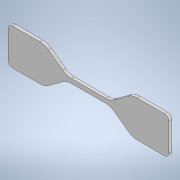
# Autodesk Inventor part: Tensile Test Specimen
Saved by Autodesk Inventor 2020 (Build 240168000, 168)
## iProperties
Created: 2020-04-08
Part Number: Tensile Test Specimen
Material: Generic
Document SubType Name: Modeling
Designer: Naude Conradie
Density: 1 g/cm^3
Appearance: Default
Author: Naude Conradie
Autodesk Inventor part; units mm, degrees
ref_plane "YZ Plane" through (0, 0, 0) normal (1, 0, 0) x (0, 1, 0)
ref_plane "XZ Plane" through (0, 0, 0) normal (0, 1, 0) x (-1, 0, 0)
ref_plane "XY Plane" through (0, 0, 0) normal (0, 0, 1) x (1, 0, 0)
sketch "Sketch1" plane through (0, 0, 0) normal (0, 0, 1) x (1, 0, 0)
  line L0 (0, 0) -> (25, 0)
  line L1 (25, 25) -> (0, 25)
  line L2 (0, 25) -> (0, 0)
  line L3 (40, 14) -> (70, 14)
  line L4 (70, 11) -> (40, 11)
  line L5 (85, 0) -> (110, 0)
  line L6 (110, 0) -> (110, 25)
  line L7 (110, 25) -> (85, 25)
  line L8 (25, 25) -> (40, 14)
  line L9 (25, 0) -> (40, 11)
  line L10 (70, 14) -> (85, 25)
  line L11 (70, 11) -> (85, 0)
  point P0 (45, 12.5)
  point P1 (25, 12.5)
  dimension "d0" = 25
  dimension "d1" = 25
  dimension "d5" = 25
  dimension "d6" = 110
  dimension "d12" = 3
  dimension "d13" = 1.5
  dimension "d14" = 30
  constraints: 24 end point, 5 equal length, 4 parallel, 3 horizontal, 2 vertical alignment, 1 horizontal alignment, 1 perpendicular
  measures "d0" distance of L1.end L1.start
  measures "d1" distance of L1.start L0.end
  measures "d5" distance of L6.end L5.end
  measures "d6" distance between parallel lines of L6 L2
  measures "d12" distance between parallel lines of L3 L4
  measures "d13" distance from line of point (45, 12.5) L3
  measures "d14" distance of L3.start L3.end
extrude "Extrusion1" add sketch "Sketch1" along normal blind 2
fillet "Fillet1" radius 10 8 edges at (25, 25, 1) (40, 14, 1) (70, 14, 1) (85, 25, 1) (25, 0, 1) (40, 11, 1) (70, 11, 1) (85, 0, 1)
fillet "Fillet2" radius 3 4 edges at (0, 25, 1) (0, 0, 1) (110, 25, 1) (110, 0, 1)
body "Solid1"
